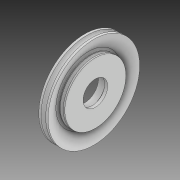
# Autodesk Inventor part: Cablecar_drivepulley
Saved by Autodesk Inventor 2020 (Build 240168000, 168)
## iProperties
Created: 2021-02-03
Part Number: Cablecar_drivepulley
Material: Generic
Document SubType Name: Modeling
Designer: DDeGo
Density: 1 g/cm^3
Appearance: Default
Author: DDeGo
Autodesk Inventor part; units mm, degrees
ref_plane "YZ Plane" through (0, 0, 0) normal (1, 0, 0) x (0, 1, 0)
ref_plane "XZ Plane" through (0, 0, 0) normal (0, 1, 0) x (-1, 0, 0)
ref_plane "XY Plane" through (0, 0, 0) normal (0, 0, 1) x (1, 0, 0)
sketch "Sketch1" plane through (0, 0, 0) normal (0, 0, 1) x (1, 0, 0)
  arc A0 (1.5, 0) -> (-1.5, 0) centre (0, 0) ccw
  line L0 (-3, 10) -> (-1, 10) construction
  line L1 (-0.4429, 8.6073) -> (3, 0)
  line L2 (3, 0) -> (1.5, 0)
  line L3 (-1.5, 0) -> (-3, 0)
  line L4 (-3, 10) -> (-3, 20.93)
  line L5 (-3, 20.93) -> (-1, 20.93)
  line L6 (-1, 20.93) -> (-1, 10) construction
  line L7 (-1, 20.93) -> (-1, 30) construction
  line L8 (-1, 30) -> (-3, 30) construction
  line L9 (-3, 30) -> (-3, 20.93) construction
  line L10 (-3, 10) -> (-3, 2)
  line L11 (-3, 2) -> (-3, 0)
  line L12 (-1, 20.93) -> (1.2, 20.93)
  line L13 (1.2, 20.93) -> (1.2, 21.93) construction
  line L14 (1.2, 21.93) -> (2.0391, 21.93) construction
  line L15 (4, 21.93) -> (4, 10)
  line L16 (4, 10) -> (3, 10)
  line L17 (3, 10) -> (1, 10) construction
  line L18 (1, 10) -> (0.5, 10)
  arc A1 (3, 10) -> (1, 10) centre (2, 10) ccw
  line L19 (1.2, 20.93) -> (2.0391, 21.93)
  line L20 (2.0391, 21.93) -> (4, 21.93)
  arc A2 (0.5, 10) -> (-0.4429, 8.6073) centre (0.5, 8.9845) ccw
  dimension "d0" = 1.5
  dimension "d1" = 2
  dimension "d2" = 6
  dimension "d4" = 9.07
  dimension "d5" = 30
  dimension "d7" = 2
  dimension "d9" = 1
  dimension "d10" = 20
  dimension "d11" = 1
  dimension "d12" = 4.2
  dimension "d13" = 1
  dimension "d15" = 5
  dimension "d16" = 40
  dimension "d17" = 1.0155
  dimension "d18" = 0.5
  constraints: 42 end point, 10 perpendicular, 8 point on line, 6 point on circle, 3 centre point, 3 coincident, 2 collinear, 2 horizontal, 2 parallel, 2 tangent, 2 vertical, 1 midpoint
  measures "d0" radius of A0
  measures "d1" distance of L0.end L0.start
  measures "d2" distance of L3.end L1.end
  measures "d4" distance between parallel lines of L5 L8
  measures "d5" distance between parallel lines of L3 L8
  measures "d7" distance of L10.end L3.end
  measures "d9" radius of A1
  measures "d10" distance between parallel lines of L8 L17
  measures "d11" distance of L15.end L16.end
  measures "d12" distance between parallel lines of L13 L9
  measures "d13" distance between parallel lines of L12 L14
  measures "d15" distance from line of point (2, 10) L4
  measures "d16" angle of L13 L19
  measures "d17" radius of A2
  measures "d18" distance of L17.end L18.end
revolve "Revolution1" add sketch "Sketch1" angle 360 about axis through (-1, 30, 0) along (-1, 0, 0)
body "Solid1"
